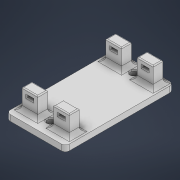
# Autodesk Inventor part: CableHolderMain
Saved by Autodesk Inventor 2022 (Build 260153000, 153)
## iProperties
Created: 2023-11-27
Part Number: CableHolderMain
Material: Všeobecné
Document SubType Name: Modeling
Designer: tada
Density: 1 g/cm^3
Appearance: Výchozí
Author: tada
Autodesk Inventor part; units mm, degrees
ref_plane "YZ Plane" through (0, 0, 0) normal (1, 0, 0) x (0, 1, 0)
ref_plane "XZ Plane" through (0, 0, 0) normal (0, 1, 0) x (-1, 0, 0)
ref_plane "XY Plane" through (0, 0, 0) normal (0, 0, 1) x (1, 0, 0)
sketch "Náčrt1" plane through (0, 0, 0) normal (0, 1, 0) x (-1, 0, 0)
  line L0 (0, 0) -> (-30, 0)
  line L1 (-30, 0) -> (-30, -55)
  line L2 (-30, -55) -> (0, -55)
  line L3 (0, -55) -> (0, 0)
  circle A0 centre (-15, -7.45) radius 1.6
  circle A1 centre (-15, -49.75) radius 1.6
  dimension "d1" = 3.2
  dimension "d2" = 3.2
  dimension "d3" = 55
  dimension "d4" = 30
  dimension "d5" = 15
  dimension "d6" = 15
  dimension "d11" = 5.25
  dimension "d12" = 7.45
  constraints: 8 end point, 2 centre point, 2 parallel, 1 horizontal, 1 perpendicular
  measures "d1" diameter of A0
  measures "d2" diameter of A1
  measures "d3" distance between parallel lines of L0 L2
  measures "d4" distance between parallel lines of L3 L1
  measures "d5" distance from line of L1 A0.centre
  measures "d6" distance from line of L1 A1.centre
  measures "d11" distance from line of L2 A1.centre
  measures "d12" distance from line of L0 A0.centre
extrude "Vysunutí1" add sketch "Náčrt1" along normal blind 3
sketch "Náčrt2" plane through (0, 3, 0) normal (0, 1, 0) x (1, 0, 0)
  line L0 (3, 5) -> (11, 5)
  line L1 (11, 5) -> (11, 10)
  line L2 (11, 10) -> (3, 10)
  line L3 (3, 10) -> (3, 5)
  line L4 (27, 5) -> (19, 5)
  line L5 (19, 5) -> (19, 10)
  line L6 (19, 10) -> (27, 10)
  line L7 (27, 10) -> (27, 5)
  line L8 (0, 55) -> (0, 0) projected
  line L9 (0, 0) -> (30, 0) projected
  line L10 (30, 0) -> (30, 55) projected
  line L11 (-2.5391, 27.5) -> (32.8549, 27.5) construction
  line L12 (3, 47.5) -> (11, 47.5)
  line L13 (11, 47.5) -> (11, 52.5)
  line L14 (11, 52.5) -> (3, 52.5)
  line L15 (3, 52.5) -> (3, 47.5)
  line L16 (19, 47.5) -> (27, 47.5)
  line L17 (27, 47.5) -> (27, 52.5)
  line L18 (27, 52.5) -> (19, 52.5)
  line L19 (19, 52.5) -> (19, 47.5)
  line L20 (30, 55) -> (0, 55) projected
  dimension "d15" = 3
  dimension "d16" = 8
  dimension "d17" = 5
  dimension "d18" = 5
  dimension "d19" = 5
  dimension "d20" = 3
  dimension "d21" = 8
  dimension "d22" = 5
  dimension "d23" = 5
  dimension "d24" = 8
  dimension "d25" = 2.5
  dimension "d26" = 2.5
  dimension "d27" = 8
  dimension "d28" = 5
  dimension "d29" = 3
  dimension "d30" = 3
  constraints: 34 end point, 8 parallel, 6 horizontal, 4 perpendicular
  measures "d15" distance between parallel lines of L8 L3
  measures "d16" distance between parallel lines of L3 L1
  measures "d17" distance between parallel lines of L2 L0
  measures "d18" distance between parallel lines of L9 L0
  measures "d19" distance between parallel lines of L9 L4
  measures "d20" distance between parallel lines of L10 L7
  measures "d21" distance between parallel lines of L5 L7
  measures "d22" distance between parallel lines of L4 L6
  measures "d23" distance between parallel lines of L14 L12
  measures "d24" distance between parallel lines of L15 L13
  measures "d25" distance between parallel lines of L20 L14
  measures "d26" distance between parallel lines of L20 L18
  measures "d27" distance between parallel lines of L17 L19
  measures "d28" distance between parallel lines of L16 L18
  measures "d29" distance between parallel lines of L8 L15
  measures "d30" distance between parallel lines of L17 L10
extrude "Vysunutí2" add sketch "Náčrt2" along normal blind 10 contours L3 L2 L1 L0 | L4 L5 L6 L7 | L15 L14 L13 L12 | L19 L18 L17 L16
fillet "Zaoblení1" radius 2 20 edges at (7, 3, -10) (23, 3, -10) (7, 3, -47.5) (23, 3, -47.5) (27, 3, -50) (23, 3, -52.5) (19, 3, -50) (11, 3, -50) (7, 3, -52.5) (3, 3, -50) (3, 3, -7.5) (7, 3, -5) (19, 3, -7.5) (23, 3, -5) (11, 3, -7.5) (27, 3, -7.5) (30, 1.5, 0) (0, 1.5, 0) (30, 1.5, -55) (0, 1.5, -55)
sketch "Náčrt3" plane through (3, 13, -5) normal (0, 0, 1) x (1, 0, 0)
  line L0 (2, -2) -> (6, -2)
  line L1 (6, -2) -> (6, -4)
  line L2 (6, -4) -> (2, -4)
  line L3 (2, -4) -> (2, -2)
  line L4 (18, -2) -> (22, -2)
  line L5 (22, -2) -> (22, -4)
  line L6 (22, -4) -> (18, -4)
  line L7 (18, -4) -> (18, -2)
  line L8 (0, -8) -> (0, 0) projected
  line L9 (0, 0) -> (8, 0) projected
  line L10 (24, -8) -> (24, 0) projected
  point P0 (-3, -13)
  dimension "d34" = 4
  dimension "d35" = 2
  dimension "d36" = 2
  dimension "d37" = 2
  dimension "d38" = 4
  dimension "d39" = 2
  dimension "d40" = 2
  constraints: 16 end point, 4 parallel, 2 horizontal, 2 perpendicular, 1 point on line
  measures "d34" distance between parallel lines of L3 L1
  measures "d35" distance between parallel lines of L8 L3
  measures "d36" distance between parallel lines of L9 L0
  measures "d37" distance between parallel lines of L0 L2
  measures "d38" distance between parallel lines of L5 L7
  measures "d39" distance between parallel lines of L4 L6
  measures "d40" distance between parallel lines of L10 L5
extrude "Vysunutí3" cut sketch "Náčrt3" against normal blind 50
fillet "Zaoblení2" radius 0.5 16 edges at (3, 13, -7.5) (7, 13, -5) (11, 13, -7.5) (7, 13, -10) (23, 13, -5) (19, 13, -7.5) (23, 13, -10) (27, 13, -7.5) (3, 13, -50) (7, 13, -52.5) (7, 13, -47.5) (11, 13, -50) (19, 13, -50) (23, 13, -52.5) (23, 13, -47.5) (27, 13, -50)
chamfer "Zkosení1" distance 0.5 angle 45 2 edges at (16.6, 3, -7.45) (16.6, 3, -49.75)
